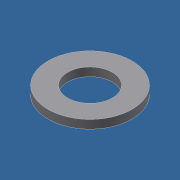
# Autodesk Inventor part: ISO7089_M5
Saved by Autodesk Inventor 2021.3 (Build 253353000, 353)
## iProperties
Created: 2022-10-02
Part Number: ISO7089_M5
Project: Visserie
Material: Acier zingué, clair
Description: Rondelles sans chanfrein
Document SubType Name: Modeling
Designer: Jean-Marc.VULLIAMY
Authority: BN715
Density: 7.85 g/cm^3
Appearance: Par défaut
Mass: 0.119485 g
Surface Area: 0.769062 cm^2
Volume: 0.015221 cm^3
Material number: ---
Author: Jean-Marc.VULLIAMY
Autodesk Inventor part; units mm, degrees
ref_plane "Plan YZ" through (0, 0, 0) normal (1, 0, 0) x (0, 1, 0)
ref_plane "Plan XZ" through (0, 0, 0) normal (0, 1, 0) x (-1, 0, 0)
ref_plane "Plan XY" through (0, 0, 0) normal (0, 0, 1) x (1, 0, 0)
sketch "Esquisse1" plane through (0, 0, 0) normal (0, 0, 1) x (1, 0, 0)
  circle A0 centre (0, 0) radius 2.65
  circle A1 centre (0, 0) radius 5
  dimension "d0" = 10
  dimension "d1" = 5.3
  constraints: 2 centre point, 2 coincident
  measures "d0" diameter of A1
  measures "d1" diameter of A0
extrude "Extrusion1" add sketch "Esquisse1" along normal blind 1
